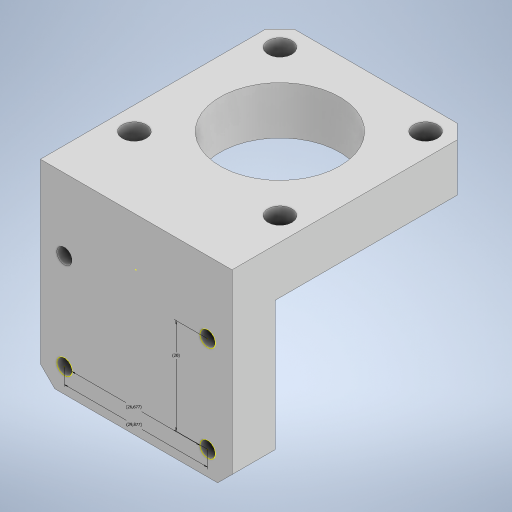
# Autodesk Inventor part: MotorMount
Saved by Autodesk Inventor 2024 (Build 280153000, 153)
## iProperties
Created: 2025-05-07
Part Number: MotorMount
Material: Generic
Document SubType Name: Modeling
Designer: Bjarni Heselmans
Density: 1 g/cm^3
Appearance: Default
Author: Bjarni Heselmans
Autodesk Inventor part; units mm, degrees
ref_plane "YZ Plane" through (0, 0, 0) normal (1, 0, 0) x (0, 1, 0)
ref_plane "XZ Plane" through (0, 0, 0) normal (0, 1, 0) x (-1, 0, 0)
ref_plane "XY Plane" through (0, 0, 0) normal (0, 0, 1) x (1, 0, 0)
sketch "Sketch1" plane through (0, 0, 0) normal (0, 0, 1) x (1, 0, 0)
  line L0 (20.0617, 19.9177) -> (20.0617, -20.0823)
  line L1 (20.0617, -20.0823) -> (-19.9383, -20.0823)
  line L2 (-19.9383, -20.0823) -> (-19.9383, 19.9177)
  line L3 (20.0617, 19.9177) -> (-19.9383, 19.9177)
  line L4 (-19.9383, 29.9177) -> (-19.9383, -30.0823)
  line L5 (15.2617, 19.9177) -> (15.2617, 15.1177)
  line L6 (15.2617, 19.9177) -> (20.0617, 19.9177) construction
  circle A0 centre (15.2617, 15.1177) radius 1.6
  line L7 (-19.9383, -0.0823) -> (20.0617, -0.0823)
  line L8 (0.0617, -20.0823) -> (0.0617, 19.9177)
  circle A1 centre (15.2617, -15.2823) radius 1.6
  circle A2 centre (-15.1383, -15.2823) radius 1.6
  circle A3 centre (-15.1383, 15.1177) radius 1.6
  arc A4 (10.0617, 7.4177) -> (10.0617, -7.5823) centre (0.0617, -0.0823) ccw
  line L9 (-12.4383, -0.0823) -> (2.0617, -0.0823)
  circle A5 centre (0.0617, -0.0823) radius 12.5
  point P0 (0, 0)
  dimension "d0" = 40
  dimension "d1" = 40
  dimension "d2" = 4.8
  dimension "d3" = 90
  dimension "d4" = 4.8
  dimension "d5" = 3.2
  dimension "d6" = 25
  dimension "d7" = 20
  dimension "d8" = 4.8
  dimension "d9" = 3.2
  dimension "d10" = 25
  dimension "d11" = 40
  dimension "d12" = 40
  constraints: 20 end point, 6 centre point, 6 midpoint, 4 point on line, 3 perpendicular, 3 point on circle, 3 symmetric about line, 2 coincident, 1 concentric, 1 horizontal, 1 parallel, 3 other
  measures "d0" distance of L0.end L2.start
  measures "d1" distance of L3.start L0.end
  measures "d2" distance of L5.start L5.end
  measures "d3" angle of L5 L6
  measures "d4" distance between parallel lines of L0 L5
  measures "d5" diameter of A0
  measures "d6" diameter of A4
  measures "d7" distance from line of A4.centre L1
  measures "d8" distance from line of L1 A1.centre
  measures "d9" diameter of A1
  measures "d10" diameter of A5
  measures "d11" diameter of L0 L8
  measures "d12" diameter of L2 L8
extrude "Extrusion1" add sketch "Sketch1" along normal blind 10 contours L0 L7 A5 A4 L8 L3 | L0 L1 L8 A4 A5 L7 | L8 A4 L7 L2 L3 | L1 L2 L7 A4 L8
sketch "Sketch2" plane through (-19.9383, -20.0823, 0) normal (0, -1, 0) x (1, 0, 0)
  line L0 (40, 0) -> (40, 10) projected
  line L1 (40, 10) -> (0, 10)
  line L2 (0, 10) -> (0, -30)
  line L3 (0, -30) -> (40, -30)
  line L4 (40, -30) -> (40, 10)
  point P0 (19.9383, 0)
  dimension "d15" = 40
  dimension "d21" = 40
  constraints: 8 end point, 2 parallel, 1 horizontal, 1 perpendicular
  measures "d15" distance of L2.end L1.end
  measures "d21" distance between parallel lines of L4 L2
extrude "Extrusion2" add sketch "Sketch2" along normal blind 10
chamfer "Chamfer1" distance 3 angle 45 2 edges at (-19.9383, 19.9177, 5) (20.0617, 19.9177, 5)
sketch "Sketch3" plane through (-19.9383, -20.0823, 0) normal (0, 1, 0) x (1, 0, 0)
  line L0 (0, 0) -> (0, 30) projected
  line L1 (0, 0) -> (5, 0)
  line L2 (5, 0) -> (5, 5)
  line L3 (5, 5) -> (0, 5)
  line L4 (0, 5) -> (0, 0)
  circle A0 centre (5, 5) radius 1.6
  line L5 (19.9383, 0) -> (19.9383, 30)
  line L6 (0, 15) -> (41.8735, 15)
  circle A1 centre (5, 25) radius 1.6
  circle A2 centre (34.8766, 5) radius 1.6
  circle A3 centre (34.8766, 25) radius 1.6
  dimension "d22" = 5
  dimension "d23" = 5
  dimension "d24" = 3.2
  constraints: 12 end point, 4 centre point, 3 symmetric about line, 2 horizontal, 2 parallel, 1 coincident, 1 midpoint, 1 perpendicular, 1 vertical, 3 other
  measures "d22" distance of L3.end L2.end
  measures "d23" distance of L2.end L1.end
  measures "d24" diameter of A0
hole "Hole1" at (-14.9383, -20.0823, -25) at (14.9383, -20.0823, -25) at (14.9383, -20.0823, -5) at (-14.9383, -20.0823, -5) direction (0, -1, 0) diameter 3.2 end through all counterbore diameter 5 counterbore depth 5
sketch "Sketch4" plane through (0, 0, 10) normal (0, 0, 1) x (1, 0, 0)
  circle A0 centre (-15.1383, 15.1177) radius 1.6 projected
  line L0 (0, 0) -> (-15.1383, 0)
  line L1 (-15.1383, 0) -> (-15.1383, 15.1177)
  line L2 (-15.1383, 15.1177) -> (0, 15.1177)
  line L3 (0, 15.1177) -> (0, 0)
  circle A1 centre (15.2617, -15.2823) radius 1.6 projected
  line L4 (-15.1383, 15.1177) -> (15.2617, 15.1177)
  line L5 (15.2617, 15.1177) -> (15.2617, -15.2823)
  line L6 (15.2617, -15.2823) -> (-15.1383, -15.2823)
  line L7 (-15.1383, -15.2823) -> (-15.1383, 15.1177)
  circle A2 centre (-15.1383, 15.1177) radius 1.6
  circle A3 centre (15.2617, 15.1177) radius 1.6 projected
  circle A4 centre (15.2617, 15.1177) radius 1.6
  circle A5 centre (15.2617, -15.2823) radius 1.6
  circle A6 centre (-15.1383, -15.2823) radius 1.6
  constraints: 16 end point, 4 centre point, 4 coincident, 4 parallel, 2 horizontal, 2 perpendicular
hole "Hole2" at (-15.1383, 15.1177, 10) at (15.2617, 15.1177, 10) at (15.2617, -15.2823, 10) at (-15.1383, -15.2823, 10) direction (0, 0, -1) diameter 3.2 end through all counterbore diameter 5 counterbore depth 5
sketch "Sketch5" plane through (-19.9383, -30.0823, 0) normal (0, -1, 0) x (1, 0, 0)
  circle A0 centre (5, -25) radius 1.6 projected
  circle A1 centre (34.8766, -25) radius 1.6 projected
  circle A2 centre (34.8766, -5) radius 1.6 projected
  point P0 (19.9383, 0)
  dimension "d39" = 26.6766
  dimension "d40" = 29.8766
  dimension "d41" = 20
  measures "d40" distance of A0.centre A1.centre
  measures "d41" distance of A2.centre A1.centre
sketch "Sketch6" plane through (-19.9383, -20.0823, 0) normal (0, 1, 0) x (1, 0, 0)
  line L0 (0, 0) -> (40, 0) projected
  line L1 (0, 30) -> (40, 30) projected
  line L2 (0, 0) -> (40, 0)
  line L3 (40, 0) -> (40, 30)
  line L4 (40, 30) -> (0, 30)
  line L5 (0, 30) -> (0, 0)
  point P0 (19.9383, 0)
  constraints: 8 end point, 2 parallel, 1 horizontal, 1 perpendicular
extrude "Extrusion3" cut sketch "Sketch6" against normal blind 1
chamfer "Chamfer2" distance 3 angle 45 2 edges at (20.0617, -25.5823, -30) (-19.9383, -25.5823, -30)
body "Solid1"
